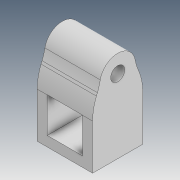
# Autodesk Inventor part: AL_PipeMount
Saved by Autodesk Inventor 2021.4 (Build 254397000, 397)
## iProperties
Created: 2022-02-25
Part Number: AL_PipeMount
Material: Generisch
Document SubType Name: Modeling
Designer: eagle
Density: 1 g/cm^3
Appearance: Vorgabe
Author: eagle
Autodesk Inventor part; units mm, degrees
ref_plane "YZ Plane" through (0, 0, 0) normal (1, 0, 0) x (0, 1, 0)
ref_plane "XZ Plane" through (0, 0, 0) normal (0, 1, 0) x (-1, 0, 0)
ref_plane "XY Plane" through (0, 0, 0) normal (0, 0, 1) x (1, 0, 0)
sketch "Skizze1" plane through (0, 0, 0) normal (0, 0, 1) x (1, 0, 0)
  line L0 (-5.275, 5.275) -> (5.275, 5.275)
  line L1 (5.275, 5.275) -> (5.275, -5.275)
  line L2 (5.275, -5.275) -> (-5.275, -5.275)
  line L3 (-5.275, -5.275) -> (-5.275, 5.275)
  line L4 (-5.275, 5.275) -> (5.275, -5.275) construction
  line L5 (5.275, 5.275) -> (-5.275, -5.275) construction
  line L6 (8.275, 8.275) -> (-8.275, 8.275)
  line L7 (-8.275, 8.275) -> (-8.275, -8.275)
  line L8 (-8.275, -8.275) -> (8.275, -8.275)
  line L9 (8.275, -8.275) -> (8.275, 8.275)
  point P0 (0, 0)
  dimension "d0" = 10.55
  dimension "d1" = 10.55
  dimension "d2" = 3
  constraints: 20 end point, 4 parallel, 2 midpoint, 2 perpendicular, 1 horizontal, 3 other
  measures "d0" distance of L1.end L2.end
  measures "d1" distance of L0.end L1.end
  measures "d2" distance between parallel lines of L0 L6
extrude "Extrusion1" add sketch "Skizze1" along normal blind 15
sketch "Skizze2" plane through (8.275, -8.275, 0) normal (1, 0, 0) x (0, 0, -1)
  line L0 (0, 0) -> (0, 16.55) projected
  line L1 (0, 16.55) -> (-15, 16.55) projected
  line L2 (-15, 0) -> (-15, 16.55) projected
  line L3 (0, 0) -> (-15, 0) projected
  circle A0 centre (-7.5, 22) radius 2.1
  circle A1 centre (-7.5, 22) radius 5.3
  line L4 (-15, 16.55) -> (-12.8, 22)
  line L5 (0, 16.55) -> (0, 0) projected
  line L6 (0, 16.55) -> (-2.2, 22)
  point P0 (0, 8.275)
  dimension "d5" = 4.2
  dimension "d6" = 22
  dimension "d7" = 7.5
  dimension "d8" = 3.2
  constraints: 4 end point, 2 centre point, 2 point on circle
  measures "d5" diameter of A0
  measures "d6" distance from line of L3 A0.centre
  measures "d7" horizontal distance of L0.start A0.centre
  measures "d8" radial gap between concentric circles of A0 A1
extrude "Extrusion2" add sketch "Skizze2" against normal up to surface (16.55 mm away) contours L1 L4 A1 L6 | A1
fillet "Rundung1" radius 15.75 4 edges at (0, 13.725, 2.2) (0, 8.275, 0) (0, 8.275, 15) (0, 13.725, 12.8)
equation "\"d1\" = d0"
